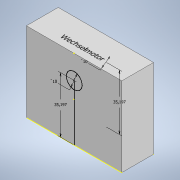
# Autodesk Inventor part: Wechselmotor
Saved by Autodesk Inventor 2021 (Build 250183000, 183)
## iProperties
Created: 2021-01-28
Part Number: Wechselmotor
Material: Generisch
Document SubType Name: Modeling
Designer: LETPJG
Density: 1 g/cm^3
Appearance: Vorgabe
Author: LETPJG
Autodesk Inventor part; units mm, degrees
ref_plane "YZ Plane" through (0, 0, 0) normal (1, 0, 0) x (0, 1, 0)
ref_plane "XZ Plane" through (0, 0, 0) normal (0, 1, 0) x (-1, 0, 0)
ref_plane "XY Plane" through (0, 0, 0) normal (0, 0, 1) x (1, 0, 0)
sketch "Skizze1" plane through (0, 0, 0) normal (0, 0, 1) x (1, 0, 0)
  line L0 (-30, 25) -> (30, 25)
  line L1 (30, 25) -> (30, -25)
  line L2 (30, -25) -> (-30, -25)
  line L3 (-30, -25) -> (-30, 25)
  line L4 (0, -25) -> (0, 10.197)
  point P0 (0, 0)
  point P1 (-30, 0)
  point P2 (0, 25)
  dimension "d0" = 60
  dimension "d1" = 50
  constraints: 10 end point, 3 midpoint, 2 parallel, 1 coincident, 1 horizontal, 1 horizontal alignment, 1 perpendicular, 1 vertical, 1 vertical alignment
  measures "d0" distance of L0.start L0.end
  measures "d1" distance of L0.end L1.end
extrude "Extrusion1" add sketch "Skizze1" against normal blind 20
sketch "Skizze2" plane through (0, 0, 0) normal (0, 0, 1) x (1, 0, 0)
  line L0 (30, -25) -> (-30, -25) projected
  line L1 (0, -25) -> (0, 10.197)
  circle A0 centre (0, 10.197) radius 5
  point P0 (0, 0)
  dimension "d6" = 35.197
  dimension "d8" = 10
  constraints: 2 coincident, 2 end point, 1 centre point, 1 midpoint, 1 vertical
  measures "d6" distance of L1.start L1.end
  measures "d8" diameter of A0
sketch "Skizze3" plane through (0, 0, -20) normal (0, 0, -1) x (-1, 0, 0)
  line L0 (-30, -25) -> (30, -25) projected
  line L1 (0, -25) -> (0, 10.197)
  circle A0 centre (0, 10.197) radius 5
  point P0 (0, 0)
  dimension "d7" = 35.197
  dimension "d9" = 10
  constraints: 2 end point, 1 centre point, 1 coincident, 1 midpoint, 1 vertical
  measures "d7" distance of L1.start L1.end
  measures "d9" diameter of A0
sketch "Skizze4" plane through (-30, 25, 0) normal (0, 1, 0) x (1, 0, 0)
  line L0 (16.6068, 7.4409) -> (69.3206, 7.4409) construction
  line L1 (69.3206, 7.4409) -> (69.3206, -2.9881) construction
  line L2 (69.3206, -2.9881) -> (16.6068, -2.9881) construction
  line L3 (16.6068, -2.9881) -> (16.6068, 7.4409) construction
  point P0 (30, 0)
  constraints: 2 other
